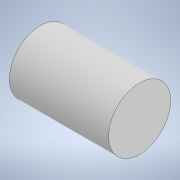
# Autodesk Inventor part: Cilindro Final diametro 20 largo 32
Saved by Autodesk Inventor 2021 (Build 250183000, 183)
## iProperties
Created: 2021-01-01
Part Number: Cilindro Final diametro 20 largo 32
Material: Generic
Document SubType Name: Modeling
Designer: dieku
Density: 1 g/cm^3
Appearance: Default
Author: dieku
Autodesk Inventor part; units mm, degrees
ref_plane "YZ Plane" through (0, 0, 0) normal (1, 0, 0) x (0, 1, 0)
ref_plane "XZ Plane" through (0, 0, 0) normal (0, 1, 0) x (-1, 0, 0)
ref_plane "XY Plane" through (0, 0, 0) normal (0, 0, 1) x (1, 0, 0)
sketch "Sketch1" plane through (0, 0, 0) normal (0, 0, 1) x (1, 0, 0)
  line L0 (0, 0) -> (0, 10)
  line L1 (0, 10) -> (32, 10)
  line L2 (32, 10) -> (32, 0)
  line L3 (32, 0) -> (0, 0)
  line L4 (0, 0) -> (43.2533, 0) construction
  dimension "d0" = 10
  dimension "d1" = 32
  constraints: 10 end point, 3 perpendicular, 1 point on line, 1 vertical
  measures "d0" distance of L0.start L0.end
  measures "d1" distance of L0.end L1.end
revolve "Revolution1" add sketch "Sketch1" angle 360 about axis through (0, 0, 0) along (1, 0, 0)
body "Solid1"
